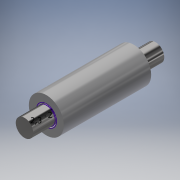
# Autodesk Inventor part: Flache Riemenscheibe1
Saved by Autodesk Inventor 2019.1 (Build 231200000, 200)
## iProperties
Created: 2018-11-28
Part Number: Flache Riemenscheibe1
Material: Steel
Document SubType Name: Modeling
Designer: JochenAlt
Density: 7.85 g/cm^3
Appearance: Steel
CustomPartVersion: 1
Author: JochenAlt
Autodesk Inventor part; units mm, degrees
ref_plane "YZ Plane" through (0, 0, 0) normal (1, 0, 0) x (0, 1, 0)
ref_plane "XZ Plane" through (0, 0, 0) normal (0, 1, 0) x (-1, 0, 0)
ref_plane "XY Plane" through (0, 0, 0) normal (0, 0, 1) x (1, 0, 0)
sketch "Hauptskizze" plane through (0, 0, 0) normal (0, 0, 1) x (1, 0, 0)
  circle A0 centre (0, 0) radius 2
  dimension "d0" = 4
  constraints: 1 centre point, 1 coincident
  measures "d0" diameter of A0
extrude "Riemenscheibe" add sketch "Hauptskizze" along normal mid plane 10
sketch "Skizze2" plane through (0, 0, 5) normal (0, 0, 1) x (1, 0, 0)
  circle A0 centre (0, 0) radius 1
  circle A1 centre (0, 0) radius 1.15
  dimension "d5" = 2
  dimension "d10" = 2.3
  constraints: 2 centre point, 2 coincident
  measures "d5" diameter of A0
  measures "d10" diameter of A1
extrude "Extrusion2" add sketch "Skizze2" along normal blind 2.5 and the other way blind 12.5 separate body contours A0
extrude "Extrusion3" cut sketch "Skizze2" against normal through all contours A0 | A1 bodies 1
equation "\"d0\" = da_D"
equation "\"d1\" = da_B"
equation "\"da_D\" = 4"
equation "\"da_B\" = 10"
body "Solid1"
